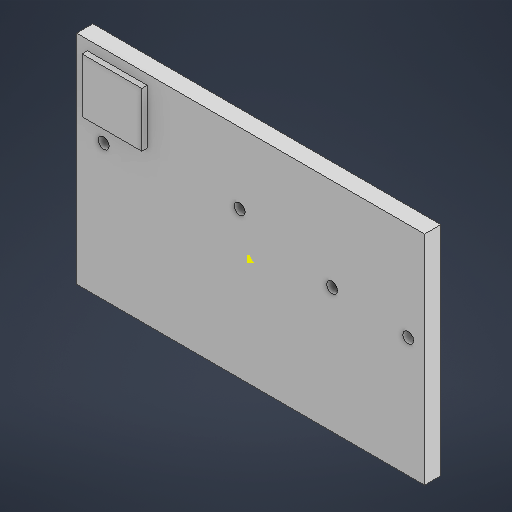
# Autodesk Inventor part: 摄像头电路部分
Saved by Autodesk Inventor 2025 (Build 290162000, 162)
## iProperties
Created: 2025-10-27
Part Number: 摄像头电路部分
Material: 常规
Document SubType Name: Modeling
Designer: XH
Density: 1 g/cm^3
Appearance: 默认
Author: XH
Autodesk Inventor part; units mm, degrees
ref_plane "YZ Plane" through (0, 0, 0) normal (1, 0, 0) x (0, 1, 0)
ref_plane "XZ Plane" through (0, 0, 0) normal (0, 1, 0) x (-1, 0, 0)
ref_plane "XY Plane" through (0, 0, 0) normal (0, 0, 1) x (1, 0, 0)
sketch "草图1" plane through (0, 0, 0) normal (0, 0, 1) x (1, 0, 0)
  line L0 (32, -20) -> (-32, -20)
  line L1 (-32, -20) -> (-32, 20)
  line L2 (-32, 20) -> (32, 20)
  line L3 (32, 20) -> (32, -20)
  line L4 (32, -20) -> (-32, 20) construction
  line L5 (-32, -20) -> (32, 20) construction
  line L6 (-32, 10) -> (-30, 10)
  line L7 (-30, 10) -> (-30, -20)
  line L8 (-30, -20) -> (-32, -20)
  line L9 (-32, -20) -> (-32, 10)
  point P0 (0, 0)
  dimension "d0" = 64
  dimension "d1" = 40
  dimension "d2" = 2
  dimension "d3" = 30
  constraints: 20 end point, 4 parallel, 2 horizontal, 2 midpoint, 2 perpendicular, 2 point on line
  measures "d0" distance of L1.end L2.end
  measures "d1" distance of L0.end L1.end
  measures "d2" distance between parallel lines of L1 L7
  measures "d3" distance between parallel lines of L0 L6
extrude "拉伸1" add sketch "草图1" along normal blind 3
sketch "草图3" plane through (0, 0, 3) normal (0, 0, 1) x (1, 0, 0)
  circle A0 centre (-27, 5) radius 1
  line L0 (-32, 20) -> (-32, -20) projected
  line L1 (32, 20) -> (-32, 20) projected
  circle A1 centre (-2, 7) radius 1
  circle A2 centre (15, 3) radius 1
  circle A3 centre (29, 2) radius 1
  line L2 (32, -20) -> (32, 20) projected
  point P0 (0, 0)
  dimension "d10" = 2
  dimension "d11" = 5
  dimension "d12" = 15
  dimension "d13" = 2
  dimension "d14" = 25
  dimension "d16" = 2
  dimension "d17" = 2
  dimension "d19" = 4
  dimension "d20" = 17
  dimension "d21" = 2
  dimension "d22" = 1
  dimension "d23" = 3
  dimension "d24" = 14
  constraints: 4 centre point
  measures "d10" diameter of A0
  measures "d11" distance from line of L0 A0.centre
  measures "d12" distance from line of A0.centre L1
  measures "d13" diameter of A1
  measures "d14" horizontal distance of A1.centre A0.centre
  measures "d16" vertical distance of A1.centre A0.centre
  measures "d17" diameter of A2
  measures "d19" vertical distance of A1.centre A2.centre
  measures "d20" horizontal distance of A1.centre A2.centre
  measures "d21" diameter of A3
  measures "d22" vertical distance of A2.centre A3.centre
  measures "d23" distance from line of A3.centre L2
  measures "d24" horizontal distance of A3.centre A2.centre
extrude "拉伸2" cut sketch "草图3" against normal blind 10
sketch "草图4" plane through (0, 0, 3) normal (0, 0, 1) x (1, 0, 0)
  line L0 (-30, 18.1876) -> (-19, 18.1876)
  line L1 (-19, 18.1876) -> (-19, 8.1876)
  line L2 (-19, 8.1876) -> (-30, 8.1876)
  line L3 (-30, 8.1876) -> (-30, 18.1876)
  line L4 (-32, 20) -> (-32, -20) projected
  point P0 (0, 0)
  dimension "d27" = 2
  dimension "d28" = 10
  dimension "d29" = 11
  constraints: 8 end point, 2 parallel, 1 horizontal, 1 perpendicular
  measures "d27" distance between parallel lines of L4 L3
  measures "d28" distance of L2.end L0.start
  measures "d29" distance of L0.start L0.end
extrude "拉伸3" add sketch "草图4" along normal blind 1
sketch "草图5" plane through (0, 0, 3) normal (0, 0, 1) x (1, 0, 0)
  point P0 (0, 0)
